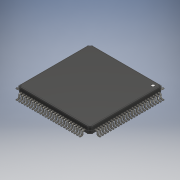
# Autodesk Inventor part: Semiconductor_QFP64-10x10
Saved by Autodesk Inventor 2018 (Build 220112000, 112)
## iProperties
Created: 2018-07-15
Part Number: Semiconductor_QFP64-10x10
Material: Generic
Document SubType Name: Modeling
Designer: Bradley
Density: 1 g/cm^3
Appearance: Smooth - Black
Author: Bradley
Autodesk Inventor part; units mm, degrees
ref_plane "YZ Plane" through (0, 0, 0) normal (1, 0, 0) x (0, 1, 0)
ref_plane "XZ Plane" through (0, 0, 0) normal (0, 1, 0) x (-1, 0, 0)
ref_plane "XY Plane" through (0, 0, 0) normal (0, 0, 1) x (1, 0, 0)
sketch "Sketch1" plane through (0, 0, 0) normal (0, 0, 1) x (1, 0, 0)
  line L0 (-6.5, -7) -> (6.5, -7)
  line L1 (7, -6.5) -> (7, 6.5)
  line L2 (6.5, 7) -> (-6.5, 7)
  line L3 (-7, 6.5) -> (-7, -6.5)
  line L4 (-7, -7) -> (7, 7) construction
  line L5 (7, -7) -> (-7, 7) construction
  line L6 (-6.5, 7) -> (-7, 6.5)
  line L7 (6.5, 7) -> (7, 6.5)
  line L8 (7, -6.5) -> (6.5, -7)
  line L9 (-7, -6.5) -> (-6.5, -7)
  point P0 (0, 0)
  dimension "d0" = 14
  dimension "d1" = 14
  dimension "d2" = 0.5
  constraints: 20 end point, 8 point on line, 5 perpendicular, 4 parallel, 2 horizontal alignment, 2 midpoint, 1 horizontal
  measures "d0" distance of L5.end L4.end
  measures "d1" distance of L4.end L5.start
  measures "d2" distance of L2.end L5.end
extrude "Extrusion1" add sketch "Sketch1" along normal mid plane 1.4 draft -10
fillet "Fillet1" radius 0.2 40 edges at (6.4744, 6.9383, 0.35) (-6.4744, 6.9383, 0.35) (0, 7, 0) (0, 6.8766, 0.7) (6.9383, 6.4744, 0.35) (6.75, 6.75, 0) (6.6627, 6.6627, 0.7) (-6.9383, 6.4744, 0.35) (-6.75, 6.75, 0) (-6.6627, 6.6627, 0.7) (6.4744, 6.9383, -0.35) (-6.4744, 6.9383, -0.35) (0, 6.8766, -0.7) (6.8766, 0, 0.7) (6.6627, -6.6627, 0.7) (0, -6.8766, 0.7) (-6.6627, -6.6627, 0.7) (-6.8766, 0, 0.7) (6.9383, -6.4744, 0.35) (7, 0, 0) (6.9383, 6.4744, -0.35) (6.6627, 6.6627, -0.7) (-6.9383, -6.4744, 0.35) (-7, 0, 0) (-6.9383, 6.4744, -0.35) (-6.6627, 6.6627, -0.7) (6.8766, 0, -0.7) (6.6627, -6.6627, -0.7) (0, -6.8766, -0.7) (-6.6627, -6.6627, -0.7) (-6.8766, 0, -0.7) (6.4744, -6.9383, 0.35) (6.75, -6.75, 0) (-6.4744, -6.9383, 0.35) (0, -7, 0) (-6.75, -6.75, 0) (6.9383, -6.4744, -0.35) (-6.9383, -6.4744, -0.35) (6.4744, -6.9383, -0.35) (-6.4744, -6.9383, -0.35)
sketch "Sketch2" plane through (0, 0, 0) normal (0, 0, 1) x (1, 0, 0)
  line L0 (7, -6.5) -> (7, 6.5) projected
  line L1 (6.5, 7) -> (-6.5, 7) projected
  line L2 (-6.5, -7) -> (6.5, -7) projected
  line L3 (7, 6.11) -> (7.3, 6.11)
  line L4 (7.3, 6.11) -> (7.3, 5.89)
  line L5 (7.3, 5.89) -> (7, 5.89)
  line L6 (7, 5.89) -> (7, 6.11)
  line L7 (7, 6.11) -> (6.7, 6.11)
  line L8 (6.7, 6.11) -> (6.7, 5.89)
  line L9 (6.7, 5.89) -> (7, 5.89)
  line L10 (7, 5.89) -> (7, 6.11)
  point P0 (0, 0)
  point P1 (7.3, 6)
  dimension "d13" = 0.22
  dimension "d14" = 6
  dimension "d15" = 0.3
  constraints: 16 end point, 4 parallel, 2 collinear, 2 horizontal, 2 perpendicular, 1 midpoint, 1 point on line
  measures "d13" distance of L3.end L4.end
  measures "d14" vertical distance of point (0, 0) point (7.3, 6)
  measures "d15" distance of L3.start L3.end
extrude "Extrusion2" add sketch "Sketch2" along normal mid plane 0.145
sketch "Sketch3" plane through (6.9872, 5.89, -0.0725) normal (0, -1, 0) x (1, 0, 0)
  line L0 (0, 0) -> (0.0067, 0.0378) projected
  line L1 (0.3128, 0) -> (0, 0) projected
  line L2 (0.3128, 0.145) -> (0.3128, 0) projected
  line L3 (0, 0.145) -> (0.3128, 0.145) projected
  line L4 (0.0067, 0.1072) -> (0, 0.145) projected
  arc A0 (0.0067, 0.0378) -> (0.0067, 0.1072) centre (-0.1903, 0.0725) ccw projected
  line L5 (0.3128, 0.145) -> (0.3128, 0) projected
  arc A1 (0.3852, -0.0681) -> (0.3128, 0) centre (0.3128, -0.0725) ccw
  line L6 (0.3852, -0.0681) -> (0.4128, -0.5232)
  arc A2 (0.4128, -0.5232) -> (0.6299, -0.7275) centre (0.6299, -0.51) ccw
  line L7 (0.6299, -0.7275) -> (1.0128, -0.7275)
  line L8 (1.0128, -0.7275) -> (1.0128, -0.5825)
  line L9 (1.0128, -0.5825) -> (0.6299, -0.5825)
  arc A3 (0.5575, -0.5144) -> (0.6299, -0.5825) centre (0.6299, -0.51) ccw
  line L10 (0.5575, -0.5144) -> (0.5299, -0.0593)
  arc A4 (0.5299, -0.0593) -> (0.3128, 0.145) centre (0.3128, -0.0725) ccw
  line L11 (0, 0.145) -> (0.3128, 0.145) projected
  line L12 (0.3128, 0) -> (0, 0) projected
  point P0 (-6.9872, 0.0725)
  dimension "d18" = 0.145
  dimension "d19" = 0.0725
  dimension "d20" = 8
  dimension "d21" = 0.8
  dimension "d22" = 0.6
  constraints: 10 end point, 8 point on circle, 7 tangent, 4 centre point, 2 concentric, 2 equal radius, 2 parallel, 1 horizontal, 1 perpendicular
  measures "d18" distance between parallel lines of L1 L3
  measures "d19" radius of A1
  measures "d20" distance from line of L8 point (-6.987, 0.072)
  measures "d21" distance from line of L7 point (-6.987, 0.072)
  measures "d22" distance from line of L6.end L8
extrude "Extrusion3" add sketch "Sketch3" against normal up to surface (0.22 mm away) contours L2 A4 L10 A3 L9 L8 L7 A2 L6 A1
pattern_linear "Rectangular Pattern1" count 25 spacing 0.5 along (0, -1, 0) of "Extrusion2", "Extrusion3"
pattern_circular "Circular Pattern1" count 4 over 360 about axis through (0, 0, -10) along (0, 0, 1) of "Extrusion2", "Extrusion3", "Rectangular Pattern1"
sketch "Sketch4" plane through (0, 0, 0.7) normal (0, 0, 1) x (1, 0, 0)
  line L0 (-6.7088, -6.3794) -> (-6.7088, 6.3794) projected
  line L1 (-6.3794, -6.7088) -> (-6.7088, -6.3794) projected
  line L2 (6.3794, -6.7088) -> (-6.3794, -6.7088) projected
  line L3 (6.7088, -6.3794) -> (6.3794, -6.7088) projected
  line L4 (6.7088, 6.3794) -> (6.7088, -6.3794) projected
  line L5 (6.3794, 6.7088) -> (6.7088, 6.3794) projected
  line L6 (-6.3794, 6.7088) -> (6.3794, 6.7088) projected
  line L7 (-6.7088, 6.3794) -> (-6.3794, 6.7088) projected
  circle A0 centre (6, 6) radius 0.25
  point P0 (0, 0)
  dimension "d31" = 0.5
  dimension "d32" = 6
  dimension "d33" = 6
  constraints: 1 centre point
  measures "d31" diameter of A0
  measures "d32" horizontal distance of A0.centre point (0, 0)
  measures "d33" horizontal distance of point (0, 0) A0.centre
extrude "Extrusion4" add sketch "Sketch4" along normal blind 0.01 contours A0
equation "\"d19\" = 0.5 * d18"
equation "\"d33\" = d32"
body "Solid1"
